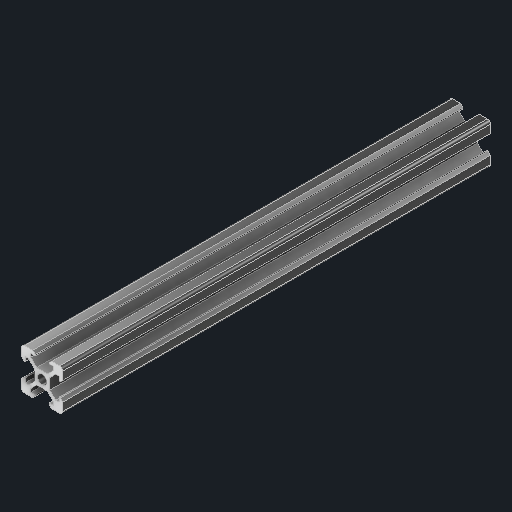
# Autodesk Inventor part: 2020aluminum_extrusion_black
Saved by Autodesk Inventor 2027.1 (Build 311270010, 270A)
## iProperties
Created: 2021-10-28
Part Number: 2020aluminum_extrusion_black
Material: Aluminum 6061
Document SubType Name: Modeling
Designer: casper
Density: 2.7 g/cm^3
Appearance: Satin - Black
Mass: 80.7582 g
Surface Area: 293.678 cm^2
Volume: 29.9105 cm^3
Author: casper
Autodesk Inventor part; units mm, degrees
ref_plane "YZ Plane" through (0, 0, 0) normal (1, 0, 0) x (0, 1, 0)
ref_plane "XZ Plane" through (0, 0, 0) normal (0, 1, 0) x (-1, 0, 0)
ref_plane "XY Plane" through (0, 0, 0) normal (0, 0, 1) x (1, 0, 0)
sketch "Sketch1" plane through (0, 0, 0) normal (0, 0, 1) x (1, 0, 0)
  line L0 (0, 3.7) -> (-2.6393, 3.7)
  line L1 (-2.6393, 3.7) -> (-5.5, 6.5607)
  line L2 (-5.5, 6.5607) -> (-5.5, 8.2)
  line L3 (-5.5, 8.2) -> (-3.395, 8.2)
  line L4 (-3.395, 8.2) -> (-3.395, 10)
  line L5 (-3.395, 10) -> (-10, 10)
  line L6 (-10, 10) -> (-10, 3.395)
  line L7 (-10, 3.395) -> (-8.2, 3.395)
  line L8 (-8.2, 3.395) -> (-8.2, 5.5)
  line L9 (-8.2, 5.5) -> (-6.5607, 5.5)
  line L10 (-6.5607, 5.5) -> (-3.7, 2.6393)
  line L11 (-3.7, 2.6393) -> (-3.7, 0)
  line L12 (0, 0) -> (-10, 10) construction
  circle A0 centre (0, 0) radius 2.3
  line L13 (-22.6601, 0) -> (65.9605, 0) projected
  line L14 (-3.7, 0) -> (0, 0)
  line L15 (0, 0) -> (0, 3.7)
  line L16 (11.2521, 18.9743) -> (53.3004, 18.9743) construction
  line L17 (53.3004, 18.9743) -> (53.3004, -5.624) construction
  line L18 (53.3004, -5.624) -> (11.2521, -5.624) construction
  line L19 (11.2521, -5.624) -> (11.2521, 18.9743) construction
  point P0 (-2.3, 0)
  point P1 (0, 2.3)
  dimension "d0" = 1.5
  dimension "d6" = 6.3
  dimension "d9" = 4.6
  dimension "d18" = 135
  dimension "d22" = 20
  dimension "d34" = 11
  dimension "d35" = 6.79
  dimension "d36" = 1.8
  constraints: 30 end point, 6 equal length, 6 perpendicular, 2 horizontal, 2 parallel, 2 vertical, 1 centre point, 1 coincident, 2 other
  measures "d0" distance between parallel lines of L1 L10
  measures "d6" distance between parallel lines of L0 L5
  measures "d9" diameter of A0
  measures "d18" angle of L13 L12
  measures "d22" diameter of L5 L14
  measures "d34" diameter of L2 L15
  measures "d35" diameter of L4 L15
  measures "d36" distance between parallel lines of L5 L3
extrude "Extrusion1" add sketch "Sketch1" along normal blind 208 contours L15 A0 L13 L11 L10 L9 L8 L7 L6 L5 L4 L3 L2 L1 L0
pattern_circular "Circular Pattern1" count 4 over 360 about axis through (0, 0, -10) along (0, 0, 1) of "Extrusion1"
chamfer "Chamfer1" distance 1.185 angle 45 8 edges at (-3.395, 10, 104) (3.395, 10, 104) (10, 3.395, 104) (10, -3.395, 104) (3.395, -10, 104) (-3.395, -10, 104) (-10, -3.395, 104) (-10, 3.395, 104)
fillet "Fillet1" radius 1.5 4 edges at (-10, 10, 104) (10, 10, 104) (-10, -10, 104) (10, -10, 104)
equation "\"GridProcutClearance\" = 3"
equation "\"GridBorderThickness\" = 5"
equation "\"GridBorderFillets\" = 7"
equation "\"GridTotalSize\" = 63"
equation "\"BaseTotalWidth\" = 652"
equation "\"BaseTotalLength\" = 912"
equation "\"DistanceBetweenGrid\" = 5"
equation "\"WorkspaceLength\" = 552"
equation "\"WorkspaceWidth\" = 417"
equation "\"WorkspaceHeight\" = 183"
equation "\"AxesBaseFillet\" = 15"
equation "\"Zaxis\" = 197"
equation "\"ProductTotalHeight\" = 45"
equation "\"VerticalStroke\" = 105"
equation "\"CylinderStroke\" = 75"
equation "\"BaseWoodThickness\" = 7"
equation "\"kerf\" = 1.5"
equation "\"Kerf\" = 0.3"
equation "\"RxThickness\" = 1.8"
body "Solid1"
